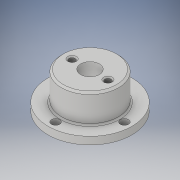
# Autodesk Inventor part: Фланецц
Saved by Autodesk Inventor 2019.3 (Build 233278000, 278)
## iProperties
Created: 2020-04-04
Part Number: Фланецц
Material: Типовые
Document SubType Name: Modeling
Designer: Admin
Density: 1 g/cm^3
Appearance: По умолчанию
Mass: 228.329 g
Surface Area: 372.967 cm^2
Volume: 228.329 cm^3
Author: Admin
Autodesk Inventor part; units mm, degrees
ref_plane "YZ Plane" through (0, 0, 0) normal (1, 0, 0) x (0, 1, 0)
ref_plane "XZ Plane" through (0, 0, 0) normal (0, 1, 0) x (-1, 0, 0)
ref_plane "XY Plane" through (0, 0, 0) normal (0, 0, 1) x (1, 0, 0)
sketch "Эскиз1" plane through (0, 0, 0) normal (0, 1, 0) x (-1, 0, 0)
  circle A0 centre (0, 0) radius 56
  dimension "d0" = 112
  constraints: 1 centre point, 1 coincident
  measures "d0" diameter of A0
extrude "Выдавливание1" add sketch "Эскиз1" along normal blind 10
sketch "Эскиз2" plane through (0, 10, 0) normal (0, 1, 0) x (1, 0, 0)
  circle A0 centre (0, 0) radius 38
  dimension "d3" = 76
  constraints: 1 centre point, 1 coincident
  measures "d3" diameter of A0
extrude "Выдавливание2" add sketch "Эскиз2" along normal blind 38
sketch "Эскиз3" plane through (0, 10, 0) normal (0, 1, 0) x (1, 0, 0)
  point P0 (0, 0)
  point P1 (-46, 0)
  dimension "d8" = 46
  constraints: 1 horizontal alignment
  measures "d8" distance of point (0, 0) point (-46, 0)
hole "Отверстие1" at (-46, 10, 0) direction (0, -1, 0) diameter 11 end through all
pattern_circular "Круговой массив1" count 4 over 360 about axis through (0, -10, 0) along (0, 1, 0) of "Отверстие1"
sketch "Эскиз4" plane through (0, 0, 0) normal (0, -1, 0) x (1, 0, 0)
  circle A0 centre (0, 0) radius 22
  dimension "d19" = 44
  constraints: 1 centre point, 1 coincident
  measures "d19" diameter of A0
extrude "Выдавливание3" cut sketch "Эскиз4" against normal blind 10
sketch "Эскиз5" plane through (0, 48, 0) normal (0, 1, 0) x (1, 0, 0)
  circle A0 centre (0, 0) radius 12.5
  dimension "d22" = 25
  constraints: 1 centre point, 1 coincident
  measures "d22" diameter of A0
extrude "Выдавливание4" cut sketch "Эскиз5" against normal through all
fillet "Сопряжение1" radius 2 1 edges at (-38, 10, 0)
chamfer "Фаска1" distance 1.6 angle 45 1 edges at (-22, 0, 0)
chamfer "Фаска2" distance 2.5 angle 45 1 edges at (-38, 48, 0)
sketch "Эскиз6" plane through (0, 48, 0) normal (0, 1, 0) x (1, 0, 0)
  point P0 (0, 0)
  point P1 (-24, 0)
  point P2 (24, 0)
  dimension "d32" = 24
  dimension "d33" = 48
  constraints: 2 horizontal alignment
  measures "d32" distance of point (0, 0) point (-24, 0)
  measures "d33" distance of point (24, 0) point (-24, 0)
hole "Отверстие2" at (-24, 48, 0) at (24, 48, 0) direction (0, -1, 0) diameter 8.376 depth 29 tip angle 120 thread size "M10x1.5" class "6H" standard "ISO Metric profile"
chamfer "Фаска3" distance 1.6 angle 45 2 edges at (-24, 48, -4.188) (24, 48, -4.188)
